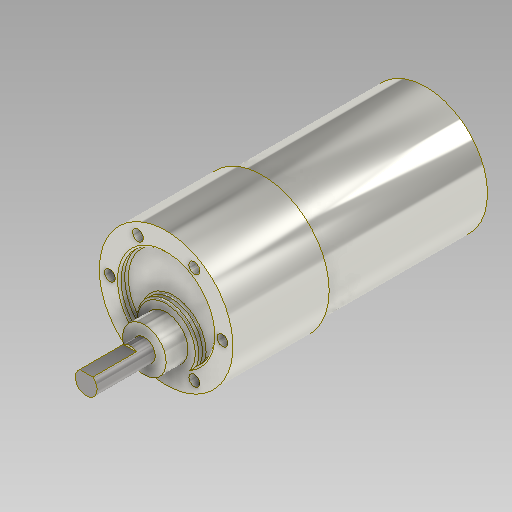
# Autodesk Inventor part: 37D mm Metal Gearbox Polulu
Saved by Autodesk Inventor 2020 (Build 240168000, 168)
## iProperties
Created: 2021-04-26
Part Number: 37D mm Metal Gearbox Polulu
Material: Stainless Steel
Document SubType Name: Modeling
Designer: Anonymus ~
Density: 8 g/cm^3
Appearance: Silver
Author: Anonymus ~
Autodesk Inventor part; units mm, degrees
ref_plane "YZ Plane" through (0, 0, 0) normal (1, 0, 0) x (0, 1, 0)
ref_plane "XZ Plane" through (0, 0, 0) normal (0, 1, 0) x (-1, 0, 0)
ref_plane "XY Plane" through (0, 0, 0) normal (0, 0, 1) x (1, 0, 0)
sketch "Sketch1" plane through (0, 0, 0) normal (0, 0, 1) x (1, 0, 0)
  circle A0 centre (0, 0) radius 18.4
  dimension "d0" = 36.8
  constraints: 1 centre point, 1 coincident
  measures "d0" diameter of A0
extrude "Extrusion1" add sketch "Sketch1" along normal blind 26.5
sketch "Sketch2" plane through (0, 0, 26.5) normal (0, 0, 1) x (1, 0, 0)
  circle A0 centre (0, -7) radius 6
  point P0 (0, 0)
  dimension "d3" = 7
  dimension "d4" = 12
  constraints: 1 centre point, 1 coincident, 1 vertical alignment
  measures "d3" distance of point (0, 0) point (0, -7)
  measures "d4" diameter of A0
extrude "Extrusion2" add sketch "Sketch2" along normal blind 6
sketch "Sketch3" plane through (0, -7, 32.5) normal (0, 0, 1) x (1, 0, 0)
  circle A0 centre (0, 0) radius 3
  point P0 (0, 7)
  dimension "d7" = 6
  constraints: 1 centre point, 1 coincident
  measures "d7" diameter of A0
extrude "Extrusion3" add sketch "Sketch3" along normal blind 16
sketch "Sketch4" plane through (0, -7, 48.5) normal (0, 0, 1) x (1, 0, 0)
  line L0 (-1.8, 2.4) -> (1.8, 2.4)
  circle A0 centre (0, 0) radius 3 projected
  point P0 (0, 7)
  dimension "d10" = 5.4
  constraints: 2 end point, 2 point on circle, 1 horizontal
extrude "Extrusion4" cut sketch "Sketch4" against normal blind 12 contours A0 L0 picked at (0, 2.6)
sketch "Sketch5" plane through (0, 0, 26.5) normal (0, 0, 1) x (1, 0, 0)
  circle A0 centre (0, 0) radius 18.4 projected
  circle A1 centre (0, 0) radius 12.9
  arc A2 (-1.8, -4.6) -> (1.8, -4.6) centre (0, -7) ccw projected
  circle A3 centre (0, -7) radius 8.5
  point P0 (-7.8641, -10.2257)
  point P1 (7.8641, -10.2257)
  dimension "d13" = 5.5
  dimension "d14" = 17
  constraints: 2 centre point, 2 coincident
  measures "d13" radial gap between concentric circles of A0 A1
  measures "d14" diameter of A3
extrude "Extrusion5" cut sketch "Sketch5" against normal blind 2 contours A1 A3 picked at (-0.0498, 9.0288)
fillet "Fillet1" radius 0.5 4 edges at (0, 12.9, 24.5) (0, 12.9, 26.5) (0, 1.5, 26.5) (0, 1.5, 24.5)
sketch "Sketch6" plane through (0, 0, 26.5) normal (0, 0, 1) x (1, 0, 0)
  circle A0 centre (-15.5, 0) radius 1.5
  circle A1 centre (-7.75, -13.4234) radius 1.5
  circle A2 centre (7.75, -13.4234) radius 1.5
  circle A3 centre (15.5, 0) radius 1.5
  circle A4 centre (7.75, 13.4234) radius 1.5
  circle A5 centre (-7.75, 13.4234) radius 1.5
  point P0 (0, 0)
  point P1 (0, 0)
  dimension "d18" = 3
  dimension "d21" = 360
  dimension "d23" = 31
  constraints: 6 centre point, 1 coincident, 1 horizontal alignment, 13 other
  measures "d18" diameter of A0
  measures "d23" distance of A3.centre A0.centre
extrude "Extrusion6" cut sketch "Sketch6" against normal through all
sketch "Sketch7" plane through (0, 0, 0) normal (0, 0, -1) x (-1, 0, 0)
  circle A0 centre (0, 0) radius 18.4
  circle A1 centre (0, 0) radius 18.4 projected
  circle A2 centre (0, 0) radius 17
  dimension "d26" = 34
  constraints: 2 centre point, 2 coincident
  measures "d26" diameter of A2
extrude "Extrusion7" add sketch "Sketch7" along normal blind 45 contours A2
body "Solid1"
